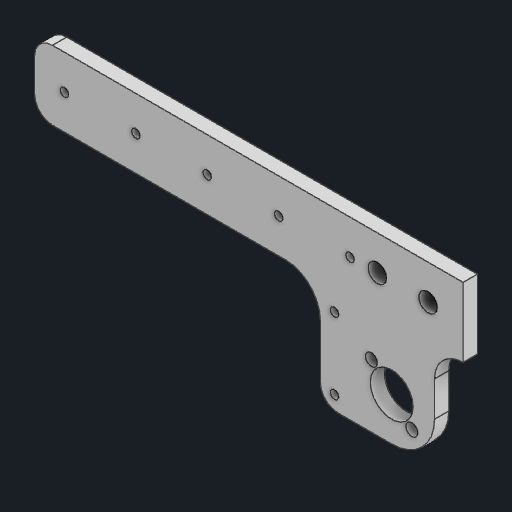
# Autodesk Inventor part: back z support
Saved by Autodesk Inventor 2024.3 (Build 283343010, 343A)
## iProperties
Created: 2024-11-30
Part Number: back z support
Material: Generic
Document SubType Name: Modeling
Designer: MFil
Density: 1 g/cm^3
Appearance: Default
Author: MFil
Autodesk Inventor part; units mm, degrees
ref_plane "YZ Plane" through (0, 0, 0) normal (1, 0, 0) x (0, 1, 0)
ref_plane "XZ Plane" through (0, 0, 0) normal (0, 1, 0) x (-1, 0, 0)
ref_plane "XY Plane" through (0, 0, 0) normal (0, 0, 1) x (1, 0, 0)
sketch "Sketch1" plane through (0, 0, 0) normal (0, 0, 1) x (1, 0, 0)
  circle A0 centre (8, 0) radius 2.6 projected
  circle A1 centre (-2, 0) radius 2.6 projected
  circle A2 centre (-12, 0) radius 2.6 projected
  line L0 (16, 9.7) -> (16, -9.7) projected
  line L1 (16, -9.7) -> (-16, -9.7) projected
  line L2 (-16, -9.7) -> (-16, 9.7) projected
  line L3 (-16, 9.7) -> (16, 9.7) projected
  circle A3 centre (-12, 0) radius 2.6 projected
  circle A4 centre (-2, 0) radius 2.6 projected
  circle A5 centre (8, 0) radius 2.6 projected
  line L4 (16, -9.7) -> (-104, -9.7)
  line L5 (-104, -9.7) -> (-104, 9.7)
  line L6 (-104, 9.7) -> (16, 9.7)
  line L7 (16, 9.7) -> (16, -9.7)
  circle A6 centre (-99, -4.7) radius 5
  line L8 (-136.5, 4.5) -> (-136.5, -4.5)
  circle A7 centre (-99, 4.7) radius 5
  point P0 (0, 0)
  point P1 (-126.8, 9.7)
  point P2 (-99, -9.7)
  point P3 (-16, -9.7)
  point P4 (-16, -9.7)
  point P5 (-104, -4.7)
  point P6 (-99, 9.7)
  point P7 (-104, 4.7)
  dimension "d0" = 120
  dimension "d1" = 19.4
  dimension "d18" = 10
  constraints: 10 end point, 4 tangent, 2 centre point, 2 parallel, 1 horizontal, 1 perpendicular, 1 vertical alignment
  measures "d0" distance of L5.end L6.end
  measures "d1" distance of L4.end L5.end
  measures "d18" diameter of A6
extrude "Extrusion1" add sketch "Sketch1" along normal blind 4 contours A0 | A1 | A2 | L0 L1 L2 L3 | L2 L4 A6 A7 L6 | A7 A6 | A6 A7 | A7 A6 L5 | A7 A6
sketch "Sketch11" plane through (0, 0, 0) normal (0, 0, -1) x (-1, 0, 0)
  circle A0 centre (-6.2, 0) radius 5
  line L0 (15, -9.7) -> (15, 9.7) projected
  circle A1 centre (8, 0) radius 5
  line L1 (-16, -9.7) -> (-16, 9.7) projected
  point P0 (0, 0)
  dimension "d109" = 10
  dimension "d110" = 10
  dimension "d111" = 9.8
  dimension "d112" = 7
  constraints: 2 centre point, 1 horizontal alignment
  measures "d109" diameter of A0
  measures "d110" diameter of A1
  measures "d111" distance from line of L1 A0.centre
  measures "d112" distance from line of L0 A1.centre
hole "Hole7" at (6.2, 0, 0) at (-8, 0, 0) direction (0, 0, 1) diameter 5.2 depth 5.5
sketch "Sketch12" plane through (0, 0, 0) normal (0, 0, -1) x (-1, 0, 0)
  circle A0 centre (15.636, 0) radius 1.75 projected
  circle A1 centre (35.636, 0) radius 1.75 projected
  circle A2 centre (55.636, 0) radius 1.75 projected
  circle A3 centre (75.636, 0) radius 1.75 projected
  circle A4 centre (95.636, 0) radius 1.75 projected
  point P0 (0, 0)
hole "Hole8" at (-15.636, 0, 0) at (-35.636, 0, 0) at (-55.636, 0, 0) at (-75.636, 0, 0) at (-95.636, 0, 0) direction (0, 0, 1) diameter 2.4 depth 5.5
sketch "Sketch13" plane through (0, 0, 0) normal (0, 0, -1) x (-1, 0, 0)
  circle A0 centre (4, -27.5001) radius 5.25 projected
  circle A1 centre (4, -27.5001) radius 12
  line L0 (-8, -27.5001) -> (-8, -17.7)
  line L1 (99, -9.7) -> (-16, -9.7) projected
  arc A2 (-8, -17.7) -> (-16, -9.7) centre (-16, -17.7) ccw
  line L2 (4, -39.5001) -> (19, -39.5001)
  arc A3 (19, -39.5001) -> (24, -34.5001) centre (19, -34.5001) ccw
  line L3 (19, -39.5001) -> (19, -34.5001) construction
  line L4 (24, -34.5001) -> (19, -34.5001) construction
  line L5 (24, -34.5001) -> (24, -19.5001)
  arc A4 (33.8001, -9.7) -> (24, -19.5001) centre (33.8001, -19.5001) ccw
  line L6 (-1.6569, -33.1569) -> (9.6569, -21.8432)
  circle A5 centre (4, -27.5001) radius 6
  point P0 (0, 0)
  dimension "d127" = 24
  dimension "d129" = 15
  dimension "d130" = 5
  dimension "d131" = 90
  dimension "d132" = 15
  dimension "d133" = 45
  dimension "d134" = 8
  dimension "d135" = 8
  dimension "d145" = 12
  constraints: 12 end point, 9 point on circle, 8 tangent, 5 centre point, 4 coincident, 2 vertical, 1 horizontal, 1 midpoint, 1 point on line
  measures "d127" diameter of A1
  measures "d129" distance of L2.start L2.end
  measures "d130" radius of A3
  measures "d131" angle of L3 L4
  measures "d132" distance of L5.start L5.end
  measures "d133" angle of L2 L6
  measures "d134" distance of A0.centre L6.start
  measures "d135" distance of A0.centre L6.end
  measures "d145" diameter of A5
extrude "Extrusion5" add sketch "Sketch13" against normal blind 4
hole "Hole9" at (1.6569, -33.1569, 0) at (-9.6569, -21.8432, 0) direction (0, 0, 1) diameter 3.4 depth 5.5
sketch "Sketch14" plane through (0, 0, 0) normal (0, 0, -1) x (-1, 0, 0)
  line L0 (24, -34.5001) -> (24, -19.5001) projected
  line L1 (4, -39.5001) -> (19, -39.5001) projected
  point P0 (0, 0)
  point P1 (20, -35.5001)
  point P2 (20, -15.5001)
  dimension "d146" = 4
  dimension "d147" = 4
  dimension "d148" = 20
  constraints: 1 vertical alignment
  measures "d146" distance from line of L0 point (20, -35.5)
  measures "d147" distance from line of L1 point (20, -35.5)
  measures "d148" distance of point (20, -35.5) point (20, -15.5)
hole "Hole10" at (-20, -35.5001, 0) at (-20, -15.5001, 0) direction (0, 0, 1) diameter 2.4 depth 5.5
equation "\"d135\" = d134"
body "Solid1"
